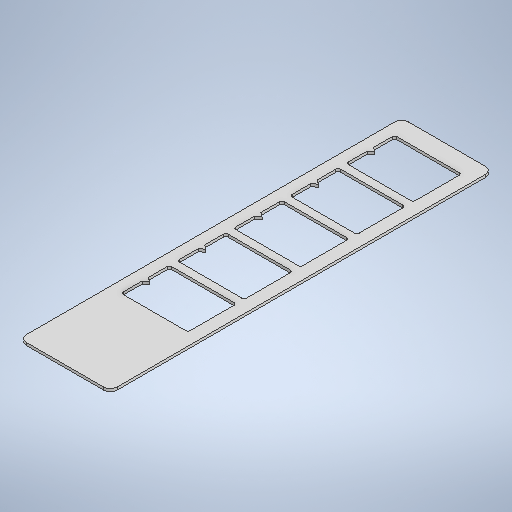
# Autodesk Inventor part: clock face
Saved by Autodesk Inventor 2025.2 (Build 292293000, 293)
## iProperties
Created: 2025-01-04
Part Number: clock face
Material: Generic
Document SubType Name: Modeling
Designer: Ian
Density: 1 g/cm^3
Appearance: Default
Author: Ian
Autodesk Inventor part; units mm, degrees
ref_plane "YZ Plane" through (0, 0, 0) normal (1, 0, 0) x (0, 1, 0)
ref_plane "XZ Plane" through (0, 0, 0) normal (0, 1, 0) x (-1, 0, 0)
ref_plane "XY Plane" through (0, 0, 0) normal (0, 0, 1) x (1, 0, 0)
sketch "Sketch1" plane through (0, 0, 0) normal (0, 1, 0) x (-1, 0, 0)
  line L0 (-4.8543, -9.3666) -> (-103.2793, -9.3666)
  line L1 (-103.2793, -9.3666) -> (-103.2793, -423.7041)
  line L2 (-103.2793, -423.7041) -> (-4.8543, -423.7041)
  line L3 (-4.8543, -423.7041) -> (-4.8543, -9.3666)
  line L4 (-103.2793, -423.7041) -> (-89.8935, -423.7041) construction
  line L5 (-103.2793, -423.7041) -> (-89.8935, -423.7041) construction
  line L6 (-89.8935, -423.7041) -> (-89.8935, -403.6381) construction
  line L7 (-89.8935, -403.6381) -> (-89.8935, -351.0601)
  line L8 (-89.8935, -351.0601) -> (-89.8935, -342.5935) construction
  line L9 (-89.8935, -342.5935) -> (-89.8935, -290.0155)
  line L10 (-89.8935, -290.0155) -> (-89.8935, -281.5488) construction
  line L11 (-89.8935, -281.5488) -> (-89.8935, -228.9708)
  line L12 (-89.8935, -228.9708) -> (-89.8935, -220.5041) construction
  line L13 (-89.8935, -220.5041) -> (-89.8935, -167.9261)
  line L14 (-89.8935, -167.9261) -> (-89.8935, -159.4595) construction
  line L15 (-89.8935, -159.4595) -> (-89.8935, -106.8815)
  line L16 (-89.8935, -403.6381) -> (-17.2495, -403.6381)
  line L17 (-17.2495, -351.0601) -> (-89.8935, -351.0601)
  line L18 (-89.8935, -342.5935) -> (-17.2495, -342.5935)
  line L19 (-17.2495, -290.0155) -> (-89.8935, -290.0155)
  line L20 (-89.8935, -281.5488) -> (-17.2495, -281.5488)
  line L21 (-17.2495, -228.9708) -> (-89.8935, -228.9708)
  line L22 (-89.8935, -220.5041) -> (-17.2495, -220.5041)
  line L23 (-17.2495, -167.9261) -> (-89.8935, -167.9261)
  line L24 (-89.8935, -159.4595) -> (-17.2495, -159.4595)
  line L25 (-17.2495, -106.8815) -> (-89.8935, -106.8815)
  line L26 (-17.2495, -373.9201) -> (-21.8723, -377.3491)
  line L27 (-17.2495, -380.7781) -> (-21.8723, -377.3491)
  line L28 (-17.2495, -319.7335) -> (-21.8723, -316.3045)
  line L29 (-17.2495, -312.8755) -> (-21.8723, -316.3045)
  line L30 (-17.2495, -258.6888) -> (-21.8723, -255.2598)
  line L31 (-17.2495, -251.8308) -> (-21.8723, -255.2598)
  line L32 (-17.2495, -190.7861) -> (-21.8723, -194.2151)
  line L33 (-17.2495, -197.6441) -> (-21.8723, -194.2151)
  line L34 (-17.2495, -136.5995) -> (-21.8723, -133.1705)
  line L35 (-17.2495, -129.7415) -> (-21.8723, -133.1705)
  line L36 (-17.2495, -403.6381) -> (-17.2495, -380.7781)
  line L37 (-17.2495, -373.9201) -> (-17.2495, -351.0601)
  line L38 (-17.2495, -342.5935) -> (-17.2495, -319.7335)
  line L39 (-17.2495, -312.8755) -> (-17.2495, -290.0155)
  line L40 (-17.2495, -281.5488) -> (-17.2495, -258.6888)
  line L41 (-17.2495, -251.8308) -> (-17.2495, -228.9708)
  line L42 (-17.2495, -220.5041) -> (-17.2495, -197.6441)
  line L43 (-17.2495, -190.7861) -> (-17.2495, -167.9261)
  line L44 (-17.2495, -159.4595) -> (-17.2495, -136.5995)
  line L45 (-17.2495, -129.7415) -> (-17.2495, -106.8815)
  point P0 (0, 0)
  dimension "d0" = 98.425
  dimension "d1" = 414.3375
  dimension "d2" = 13.3858
  dimension "d4" = 20.066
  dimension "d5" = 52.578
  dimension "d6" = 8.4667
  dimension "d7" = 52.578
  dimension "d8" = 8.4667
  dimension "d9" = 52.578
  dimension "d10" = 8.4667
  dimension "d11" = 52.578
  dimension "d12" = 8.4667
  dimension "d13" = 52.578
  dimension "d16" = 72.644
  constraints: 92 end point, 14 perpendicular, 13 parallel, 5 point on line, 3 horizontal, 3 vertical, 2 collinear
  measures "d0" distance of L2.end L1.end
  measures "d1" distance of L1.end L0.end
  measures "d2" distance of L1.end L4.end
  measures "d4" distance of L5.end L6.end
  measures "d5" distance of L6.end L7.end
  measures "d6" distance of L7.end L8.end
  measures "d7" distance of L8.end L9.end
  measures "d8" distance of L9.end L10.end
  measures "d9" distance of L10.end L11.end
  measures "d10" distance of L11.end L12.end
  measures "d11" distance of L12.end L13.end
  measures "d12" distance of L13.end L14.end
  measures "d13" distance of L14.end L15.end
  measures "d16" distance of L6.end L16.end
extrude "Extrusion1" add sketch "Sketch1" along normal blind 2.8956
fillet "Fillet1" radius 2.54 20 edges at (17.2495, 1.4478, -106.8815) (17.2495, 1.4478, -159.4595) (17.2495, 1.4478, -167.9261) (17.2495, 1.4478, -228.9708) (17.2495, 1.4478, -290.0155) (17.2495, 1.4478, -351.0601) (17.2495, 1.4478, -403.6381) (17.2495, 1.4478, -342.5935) (17.2495, 1.4478, -281.5488) (17.2495, 1.4478, -220.5041) (89.8935, 1.4478, -403.6381) (89.8935, 1.4478, -342.5935) (89.8935, 1.4478, -281.5488) (89.8935, 1.4478, -220.5041) (89.8935, 1.4478, -159.4595) (89.8935, 1.4478, -106.8815) (89.8935, 1.4478, -167.9261) (89.8935, 1.4478, -228.9708) (89.8935, 1.4478, -290.0155) (89.8935, 1.4478, -351.0601)
fillet "Fillet2" radius 7.62 4 edges at (4.8543, 1.4478, -9.3666) (103.2793, 1.4478, -9.3666) (4.8543, 1.4478, -423.7041) (103.2793, 1.4478, -423.7041)
body "Solid1"
